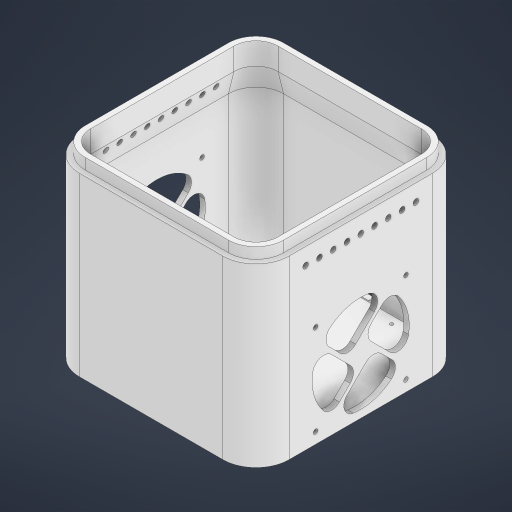
# Autodesk Inventor part: bottom part v2
Saved by Autodesk Inventor 2024.1 (Build 281209000, 209)
## iProperties
Created: 2023-07-11
Part Number: bottom part v2
Material: 일반
Document SubType Name: Modeling
Designer: 6gioc
Density: 1 g/cm^3
Appearance: 기본값
Author: 6gioc
## iProperties of the stored document bottom part v2_3D 인쇄.ipt
Created: 2023-11-02
Part Number: bottom part v2_3D 인쇄
Material: 일반
Document SubType Name: Modeling
Designer: 6gioc
Density: 1 g/cm^3
Appearance: 기본값
Author: 6gioc
Autodesk Inventor part; units mm, degrees
ref_plane "YZ Plane" through (0, 0, 0) normal (1, 0, 0) x (0, 1, 0)
ref_plane "XZ Plane" through (0, 0, 0) normal (0, 1, 0) x (-1, 0, 0)
ref_plane "XY Plane" through (0, 0, 0) normal (0, 0, 1) x (1, 0, 0)
sketch "스케치1" plane through (0, 0, 0) normal (0, 1, 0) x (-1, 0, 0)
  line L0 (-30, 0) -> (-160, 0)
  line L1 (-190, -30) -> (-190, -160)
  line L2 (-160, -190) -> (-30, -190)
  line L3 (0, -160) -> (0, -30)
  arc A0 (-30, -190) -> (0, -160) centre (-30, -160) ccw
  arc A1 (-190, -160) -> (-160, -190) centre (-160, -160) ccw
  arc A2 (-160, 0) -> (-190, -30) centre (-160, -30) ccw
  arc A3 (0, -30) -> (-30, 0) centre (-30, -30) ccw
  line L4 (-30, -185) -> (-160, -185)
  arc A4 (-185, -160) -> (-160, -185) centre (-160, -160) ccw
  line L5 (-185, -160) -> (-185, -30)
  arc A5 (-160, -5) -> (-185, -30) centre (-160, -30) ccw
  line L6 (-160, -5) -> (-30, -5)
  arc A6 (-5, -30) -> (-30, -5) centre (-30, -30) ccw
  line L7 (-5, -30) -> (-5, -160)
  arc A7 (-30, -185) -> (-5, -160) centre (-30, -160) ccw
  point P0 (0, 0)
  point P1 (-190, -190)
  point P2 (-190, 0)
  point P3 (0, -190)
  dimension "d0" = 190
  dimension "d1" = 190
  dimension "d2" = 30
  dimension "d3" = 5
  constraints: 16 end point, 16 point on circle, 8 centre point, 8 point on line, 8 tangent, 4 parallel, 3 equal radius, 2 perpendicular, 1 horizontal, 7 other
  measures "d0" distance of point (0, -190) point (-190, -190)
  measures "d1" distance of point (-190, -190) point (-190, 0)
  measures "d2" radius of A0
  measures "d3" distance between parallel lines of L2 L4
extrude "돌출1" add sketch "스케치1" along normal blind 160
extrude "돌출2" add sketch "스케치1" along normal blind 5 contours L4 A4 L5 A5 L6 A6 L7 A7
sketch "스케치2" plane through (0, 160, 0) normal (0, 1, 0) x (1, 0, 0)
  arc A0 (160, 0) -> (190, 30) centre (160, 30) ccw projected
  line L0 (190, 30) -> (190, 160) projected
  arc A1 (190, 160) -> (160, 190) centre (160, 160) ccw projected
  line L1 (160, 190) -> (30, 190) projected
  arc A2 (30, 190) -> (0, 160) centre (30, 160) ccw projected
  line L2 (0, 160) -> (0, 30) projected
  arc A3 (0, 30) -> (30, 0) centre (30, 30) ccw projected
  line L3 (30, 0) -> (160, 0) projected
  line L4 (5, 30) -> (5, 160) projected
  arc A4 (30, 185) -> (5, 160) centre (30, 160) ccw projected
  line L5 (30, 185) -> (160, 185) projected
  arc A5 (185, 160) -> (160, 185) centre (160, 160) ccw projected
  line L6 (185, 160) -> (185, 30) projected
  arc A6 (160, 5) -> (185, 30) centre (160, 30) ccw projected
  line L7 (160, 5) -> (30, 5) projected
  arc A7 (5, 30) -> (30, 5) centre (30, 30) ccw projected
  line L8 (10, 160) -> (10, 30)
  arc A8 (10, 30) -> (30, 10) centre (30, 30) ccw
  line L9 (30, 10) -> (160, 10)
  arc A9 (160, 10) -> (180, 30) centre (160, 30) ccw
  line L10 (180, 30) -> (180, 160)
  arc A10 (180, 160) -> (160, 180) centre (160, 160) ccw
  line L11 (160, 180) -> (30, 180)
  arc A11 (30, 180) -> (10, 160) centre (30, 160) ccw
  point P0 (0, 0)
  dimension "d8" = 5
  constraints: 8 end point, 8 point on circle, 4 centre point, 7 other
  measures "d8" distance between parallel lines of L4 L8
extrude "돌출3" add sketch "스케치2" along normal blind 10 contours L4 A4 L5 A5 L6 A6 L7 A7
extrude "돌출4" add sketch "스케치2" against normal blind 10 contours L4 A4 L5 A5 L6 A6 L7 A7
chamfer "모따기1" distance 5 distance2 20 8 edges at (95, 150, -5) (177.6777, 150, -12.3223) (185, 150, -95) (177.6777, 150, -177.6777) (95, 150, -185) (12.3223, 150, -177.6777) (5, 150, -95) (12.3223, 150, -12.3223) measured on face at (177.3241, 150, -12.6759) measured on face at (12.6759, 150, -177.3241) measured on face at (12.6759, 150, -12.6759) measured on face at (95, 150, -184.5) measured on face at (184.5, 150, -95) measured on face at (5.5, 150, -95) measured on face at (95, 150, -5.5) measured on face at (177.3241, 150, -177.3241)
sketch "스케치4" plane through (160, 0, -190) normal (0, 0, -1) x (-1, 0, 0)
  line L0 (53, 39.5) -> (77, 39.5)
  line L1 (80, 36.5) -> (80, 9)
  line L2 (77, 6) -> (53, 6)
  line L3 (50, 9) -> (50, 36.5)
  arc A0 (77, 6) -> (80, 9) centre (77, 9) ccw
  arc A1 (50, 9) -> (53, 6) centre (53, 9) ccw
  arc A2 (53, 39.5) -> (50, 36.5) centre (53, 36.5) ccw
  arc A3 (80, 36.5) -> (77, 39.5) centre (77, 36.5) ccw
  line L4 (0, 0) -> (130, 0) projected
  line L5 (130, 0) -> (130, 160) projected
  line L6 (0, 0) -> (0, 160) projected
  circle A4 centre (47.05, 21.1) radius 1.65
  circle A5 centre (82.95, 21.1) radius 1.65
  point P0 (160, 0)
  point P1 (80, 6)
  point P2 (80, 39.5)
  point P3 (50, 6)
  point P4 (50, 22.75)
  dimension "d16" = 30
  dimension "d17" = 33.5
  dimension "d18" = 3
  dimension "d19" = 6
  dimension "d20" = 50
  dimension "d21" = 50
  dimension "d22" = 3.3
  dimension "d23" = 3.3
  dimension "d24" = 15.1
  dimension "d25" = 35.9
  dimension "d26" = 2.95
  constraints: 8 end point, 8 point on circle, 8 tangent, 6 centre point, 6 point on line, 3 equal radius, 2 parallel, 1 horizontal, 1 horizontal alignment, 1 midpoint, 1 perpendicular
  measures "d16" distance of point (80, 6) point (50, 6)
  measures "d17" distance of point (80, 39.5) point (80, 6)
  measures "d18" radius of A0
  measures "d19" distance between parallel lines of L4 L2
  measures "d20" distance between parallel lines of L5 L1
  measures "d21" distance from line of L6 point (50, 22.75)
  measures "d22" diameter of A4
  measures "d23" diameter of A5
  measures "d24" distance from line of L2 A4.centre
  measures "d25" distance of A5.centre A4.centre
  measures "d26" distance from line of L3 A4.centre
extrude "돌출5" cut sketch "스케치4" against normal blind 10
sketch "스케치5" plane through (190, 0, -30) normal (1, 0, 0) x (0, 0, -1)
  circle A0 centre (24, 10) radius 2
  circle A1 centre (106, 10) radius 2
  circle A2 centre (106, 92) radius 2
  circle A3 centre (24, 92) radius 2
  line L0 (19, 97) -> (111, 97)
  line L1 (111, 97) -> (111, 5)
  line L2 (111, 5) -> (19, 5)
  line L3 (19, 5) -> (19, 97)
  line L4 (130, 0) -> (130, 160) projected
  line L5 (0, 0) -> (130, 0) projected
  circle A4 centre (65, 51) radius 44
  circle A5 centre (65, 51) radius 10
  line L6 (24, 92) -> (106, 10)
  line L7 (24, 10) -> (106, 92)
  line L8 (57.9289, 58.0711) -> (88.2274, 88.3696)
  line L9 (72.0711, 58.0711) -> (102.3696, 27.7726)
  line L10 (72.0711, 43.9289) -> (41.7726, 13.6304)
  line L11 (57.9289, 43.9289) -> (27.6304, 74.2274)
  line L12 (60.4038, 46.4038) -> (29.6325, 77.1751)
  line L13 (60.4038, 55.5962) -> (91.1751, 86.3675)
  line L14 (69.5962, 55.5962) -> (100.3675, 24.8249)
  line L15 (69.5962, 46.4038) -> (38.8249, 15.6325)
  circle A6 centre (65, 145) radius 2.5
  line L16 (0, 160) -> (130, 160) projected
  line L17 (130, 130) -> (0, 130) projected
  circle A7 centre (90, 145) radius 2.5
  circle A8 centre (115, 145) radius 2.5
  circle A9 centre (40, 145) radius 2.5
  circle A10 centre (15, 145) radius 2.5
  line L18 (0, 0) -> (0, 160) projected
  circle A11 centre (27.5, 145) radius 2.5
  circle A12 centre (52.5, 145) radius 2.5
  circle A13 centre (77.5, 145) radius 2.5
  circle A14 centre (102.5, 145) radius 2.5
  point P0 (-30, 0)
  point P1 (65.7774, 60.9697)
  point P2 (74.9697, 50.2226)
  point P3 (64.2226, 41.0303)
  point P4 (55.0303, 51.7774)
  point P5 (65, 145)
  dimension "d41" = 88
  dimension "d29" = 4
  dimension "d30" = 4
  dimension "d31" = 4
  dimension "d32" = 4
  dimension "d33" = 82
  dimension "d34" = 82
  dimension "d35" = 92
  dimension "d36" = 92
  dimension "d37" = 5
  dimension "d38" = 5
  dimension "d39" = 19
  dimension "d40" = 5
  dimension "d42" = 20
  dimension "d43" = 3.5
  dimension "d44" = 3.5
  dimension "d45" = 3.5
  dimension "d46" = 3.5
  dimension "d49" = 5
  dimension "d50" = 15
  dimension "d51" = 5
  dimension "d52" = 5
  dimension "d53" = 5
  dimension "d54" = 5
  dimension "d55" = 25
  dimension "d56" = 25
  dimension "d57" = 25
  dimension "d58" = 25
  dimension "d59" = 15
  dimension "d142" = 5
  dimension "d143" = 5
  dimension "d144" = 5
  dimension "d145" = 5
  dimension "d146" = 12.5
  dimension "d147" = 12.5
  dimension "d148" = 12.5
  dimension "d149" = 12.5
  constraints: 28 end point, 14 centre point, 6 horizontal alignment, 6 parallel, 4 perpendicular, 4 point on circle, 4 point on line, 4 tangent, 2 vertical alignment, 1 coincident, 1 horizontal, 21 other
  measures "d29" diameter of A0
  measures "d30" diameter of A1
  measures "d31" diameter of A2
  measures "d32" diameter of A3
  measures "d33" distance of L7.end L6.start
  measures "d34" distance of L7.start L6.start
  measures "d35" distance of L1.end L2.end
  measures "d36" distance of L0.end L1.end
  measures "d37" distance from line of L3 L6.start
  measures "d38" distance from line of L0 L6.start
  measures "d39" distance between parallel lines of L4 L1
  measures "d40" distance between parallel lines of L5 L2
  measures "d42" diameter of A5
  measures "d43" distance between parallel lines of L11 L12
  measures "d44" distance between parallel lines of L8 L13
  measures "d45" distance between parallel lines of L9 L14
  measures "d46" distance between parallel lines of L10 L15
  measures "d49" diameter of A6
  measures "d50" distance from line of L16 A6.centre
  measures "d51" diameter of A7
  measures "d52" diameter of A8
  measures "d53" diameter of A9
  measures "d54" diameter of A10
  measures "d55" distance of A6.centre A9.centre
  measures "d56" distance of A7.centre A6.centre
  measures "d57" distance of A8.centre A7.centre
  measures "d58" distance of A9.centre A10.centre
  measures "d59" distance from line of L18 A10.centre
  measures "d142" diameter of A11
  measures "d143" diameter of A12
  measures "d144" diameter of A13
  measures "d145" diameter of A14
  measures "d146" distance of A9.centre A11.centre
  measures "d147" distance of A12.centre A9.centre
  measures "d148" distance of A13.centre A6.centre
  measures "d149" distance of A8.centre A14.centre
extrude "돌출6" cut sketch "스케치5" against normal blind 5 contours A0 | A1 | A2 | A3 | A4 L7 A5 L13 | L8 L6 A4 | A4 L9 L7 | L6 A5 L12 A4 | L11 L7 A4 | A5 L15 A4 L7 | A4 L6 A5 L14 | A4 L10 L6
extrude "돌출7" cut sketch "스케치5" against normal blind 241.25 contours A6 | A7 | A8 | A9 | A10 | A11 | A12 | A13 | A14
sketch "스케치6" plane through (0, 0, -160) normal (-1, 0, 0) x (0, 0, 1)
  circle A0 centre (24, 10) radius 2
  circle A1 centre (106, 10) radius 2
  circle A2 centre (106, 92) radius 2
  circle A3 centre (24, 92) radius 2
  line L0 (19, 97) -> (111, 97)
  line L1 (111, 97) -> (111, 5)
  line L2 (111, 5) -> (19, 5)
  line L3 (19, 5) -> (19, 97)
  circle A4 centre (65, 51) radius 44
  circle A5 centre (65, 51) radius 10
  line L4 (24, 92) -> (106, 10)
  line L5 (24, 10) -> (106, 92)
  line L6 (57.9289, 58.0711) -> (88.2274, 88.3696)
  line L7 (72.0711, 58.0711) -> (102.3696, 27.7726)
  line L8 (72.0711, 43.9289) -> (41.7726, 13.6304)
  line L9 (57.9289, 43.9289) -> (27.6304, 74.2274)
  line L10 (65.7774, 60.9697) -> (91.1751, 86.3675)
  line L11 (87.4105, 64.2181) -> (38.8249, 15.6325)
  line L12 (55.0303, 51.7774) -> (29.6325, 77.1751)
  line L13 (130, 0) -> (130, 160) projected
  line L14 (0, 0) -> (130, 0) projected
  line L15 (69.5962, 55.5962) -> (100.3675, 24.8249)
  point P0 (160, 0)
  point P1 (80.7926, 9.9318)
  point P2 (64.2226, 41.0303)
  point P3 (74.9697, 50.2226)
  dimension "d72" = 88
  dimension "d62" = 4
  dimension "d63" = 4
  dimension "d64" = 4
  dimension "d65" = 4
  dimension "d66" = 82
  dimension "d67" = 82
  dimension "d68" = 92
  dimension "d69" = 92
  dimension "d70" = 5
  dimension "d71" = 5
  dimension "d73" = 20
  dimension "d75" = 3.5
  dimension "d77" = 3.5
  dimension "d78" = 3.5
  dimension "d79" = 19
  dimension "d80" = 5
  dimension "d81" = 3.5
  constraints: 28 end point, 6 parallel, 6 point on circle, 5 centre point, 4 perpendicular, 4 point on line, 4 tangent, 2 horizontal alignment, 2 vertical alignment, 1 coincident, 1 horizontal, 11 other
  measures "d62" diameter of A0
  measures "d63" diameter of A1
  measures "d64" diameter of A2
  measures "d65" diameter of A3
  measures "d66" distance of L5.end L4.start
  measures "d67" distance of L5.start L4.start
  measures "d68" distance of L1.end L3.start
  measures "d69" distance of L0.end L1.end
  measures "d70" distance from line of L3 L4.start
  measures "d71" distance from line of L0 L4.start
  measures "d73" diameter of A5
  measures "d75" distance between parallel lines of L6 L10
  measures "d77" distance between parallel lines of L8 L11
  measures "d78" distance between parallel lines of L9 L12
  measures "d79" distance between parallel lines of L13 L1
  measures "d80" distance between parallel lines of L14 L2
  measures "d81" distance between parallel lines of L7 L15
extrude "돌출8" cut sketch "스케치6" against normal blind 5 contours A0 | A1 | A2 | A3 | A4 L5 A5 L10 | L6 L4 A4 | A4 L7 L5 | L4 A5 L12 A4 | L9 L5 A4 | A5 L11 A4 L5 | A4 L4 A5 L15 | L4 A4 L8
sketch "스케치7" plane through (0, 0, 0) normal (0, -1, 0) x (1, 0, 0)
  circle A0 centre (135, -178) radius 1.5
  line L0 (160, -190) -> (30, -190) projected
  circle A1 centre (135, -104.3) radius 1.5
  circle A2 centre (147, -92.3) radius 1.5
  line L1 (190, -30) -> (190, -160) projected
  circle A3 centre (53, -178) radius 1.5
  circle A4 centre (53, -104.3) radius 1.5
  circle A5 centre (65, -92.3) radius 1.5
  line L2 (0, -160) -> (0, -30) projected
  point P0 (0, 0)
  dimension "d84" = 3
  dimension "d85" = 12
  dimension "d86" = 3
  dimension "d87" = 73.7
  dimension "d88" = 3
  dimension "d89" = 12
  dimension "d90" = 12
  dimension "d91" = 55
  dimension "d94" = 3
  dimension "d95" = 3
  dimension "d96" = 3
  dimension "d97" = 12
  dimension "d98" = 12
  dimension "d99" = 73.7
  dimension "d100" = 65
  constraints: 6 centre point, 2 vertical alignment, 1 horizontal alignment
  measures "d84" diameter of A0
  measures "d85" distance from line of L0 A0.centre
  measures "d86" diameter of A1
  measures "d87" distance of A1.centre A0.centre
  measures "d88" diameter of A2
  measures "d89" horizontal distance of A2.centre A1.centre
  measures "d90" horizontal distance of A2.centre A1.centre
  measures "d91" distance from line of L1 A0.centre
  measures "d94" diameter of A3
  measures "d95" diameter of A4
  measures "d96" diameter of A5
  measures "d97" horizontal distance of A4.centre A5.centre
  measures "d98" horizontal distance of A5.centre A4.centre
  measures "d99" distance of A4.centre A3.centre
  measures "d100" distance from line of L2 A5.centre
extrude "돌출9" cut sketch "스케치7" against normal blind 5
sketch "스케치9" plane through (0, 5, 0) normal (0, 1, 0) x (1, 0, 0)
  line L0 (185, 160) -> (185, 30) projected
  line L1 (185, 45) -> (5, 45)
  line L2 (5, 30) -> (5, 160) projected
  line L3 (185, 45) -> (365, 45) construction
  circle A0 centre (65, 92.3) radius 1.5 projected
  circle A1 centre (147, 92.3) radius 1.5 projected
  circle A2 centre (53, 104.3) radius 1.5 projected
  circle A3 centre (135, 178) radius 1.5 projected
  circle A4 centre (135, 104.3) radius 1.5 projected
  circle A5 centre (53, 178) radius 1.5 projected
  line L4 (160, 5) -> (30, 5) projected
  arc A6 (160, 5) -> (185, 30) centre (160, 30) ccw projected
  line L5 (185, 160) -> (185, 30) projected
  arc A7 (185, 160) -> (160, 185) centre (160, 160) ccw projected
  line L6 (30, 185) -> (160, 185) projected
  arc A8 (30, 185) -> (5, 160) centre (30, 160) ccw projected
  line L7 (5, 30) -> (5, 160) projected
  arc A9 (5, 30) -> (30, 5) centre (30, 30) ccw projected
  circle A10 centre (180, 40) radius 1.5
  circle A11 centre (180, 40) radius 2.5
  circle A12 centre (180, 27) radius 2.5
  circle A13 centre (163, 10) radius 1.5
  circle A14 centre (163, 10) radius 2.5
  line L8 (95, 45) -> (95, 5)
  circle A15 centre (95, 10) radius 2.5
  circle A16 centre (95, 40) radius 2.5
  circle A17 centre (137.5, 40) radius 2.5
  circle A18 centre (10, 40) radius 1.5
  circle A19 centre (10, 40) radius 2.5
  circle A20 centre (10, 27) radius 2.5
  circle A21 centre (27, 10) radius 1.5
  circle A22 centre (27, 10) radius 2.5
  circle A23 centre (52.5, 40) radius 2.5
  point P0 (0, 0)
  dimension "d108" = 180
  dimension "d109" = 40
  dimension "d110" = 3
  dimension "d111" = 5
  dimension "d112" = 5
  dimension "d113" = 3
  dimension "d114" = 5
  dimension "d115" = 5
  dimension "d116" = 5
  dimension "d117" = 5
  dimension "d118" = 5
  dimension "d119" = 5
  dimension "d121" = 5
  dimension "d122" = 3
  dimension "d123" = 5
  dimension "d124" = 5
  dimension "d125" = 5
  dimension "d126" = 5
  dimension "d127" = 42.5
  dimension "d128" = 85
  dimension "d134" = 3
  constraints: 14 centre point, 6 end point, 6 symmetric about line, 4 coincident, 4 point on line, 2 midpoint, 1 collinear, 1 horizontal, 6 other
  measures "d108" angle of L1 L3
  measures "d109" distance from line of L4 L1.start
  measures "d110" diameter of A10
  measures "d111" diameter of A11
  measures "d112" diameter of A12
  measures "d113" diameter of A13
  measures "d114" diameter of A14
  measures "d115" diameter of A15
  measures "d116" diameter of A16
  measures "d117" distance from line of L4 A15.centre
  measures "d118" distance from line of L1 A16.centre
  measures "d119" distance from line of L4 A14.centre
  measures "d121" distance from line of L0 A12.centre
  measures "d122" vertical distance of L0.end A12.centre
  measures "d123" distance from line of L0 A11.centre
  measures "d124" distance from line of L1 A11.centre
  measures "d125" diameter of A17
  measures "d126" distance from line of L1 A17.centre
  measures "d127" distance of A11.centre A17.centre
  measures "d128" distance from line of L8 A11.centre
  measures "d134" horizontal distance of L4.start A14.centre
extrude "돌출11" add sketch "스케치9" along normal blind 5 contours A16 L8 | L8 A16 | A15 L8 | L8 A15 | A11 | A12 | A14 | A17 | A19 | A20 | A22 | A23
extrude "돌출12" cut sketch "스케치9" against normal blind 5 contours A10 | A13 | A18 | A21
sketch "스케치10" plane through (0, 0, 0) normal (0, -1, 0) x (1, 0, 0)
  circle A0 centre (95, -95) radius 60
  circle A1 centre (95, -95) radius 70
  circle A2 centre (10, -40) radius 1.5 projected
  circle A3 centre (163, -10) radius 1.5 projected
  circle A4 centre (27, -10) radius 1.5 projected
  circle A5 centre (180, -40) radius 1.5 projected
  circle A6 centre (65, -92.3) radius 1.5 projected
  circle A7 centre (147, -92.3) radius 1.5 projected
  circle A8 centre (53, -104.3) radius 1.5 projected
  circle A9 centre (135, -178) radius 1.5 projected
  circle A10 centre (135, -104.3) radius 1.5 projected
  circle A11 centre (53, -178) radius 1.5 projected
  arc A12 (190, -30) -> (160, 0) centre (160, -30) ccw projected
  line L0 (30, 0) -> (160, 0) projected
  arc A13 (30, 0) -> (0, -30) centre (30, -30) ccw projected
  line L1 (0, -160) -> (0, -30) projected
  arc A14 (0, -160) -> (30, -190) centre (30, -160) ccw projected
  line L2 (160, -190) -> (30, -190) projected
  arc A15 (160, -190) -> (190, -160) centre (160, -160) ccw projected
  line L3 (190, -30) -> (190, -160) projected
  point P0 (0, 0)
  point P1 (190, -95)
  point P2 (95, 0)
  dimension "d135" = 120
  dimension "d136" = 140
  constraints: 2 centre point, 2 midpoint, 1 concentric, 1 horizontal alignment, 1 vertical alignment
  measures "d135" diameter of A0
  measures "d136" diameter of A1
extrude "돌출13" add sketch "스케치10" along normal blind 10 contours A1
chamfer "모따기2" distance 10 angle 45 1 edges at (25, 0, -95)
fillet "모깎기1" radius 10 12 edges at (2.5, 86.3675, -68.8249) (2.5, 88.3696, -71.7726) (2.5, 24.8249, -59.6325) (2.5, 15.6325, -121.1751) (2.5, 60.9697, -94.2226) (2.5, 77.1751, -130.3675) (2.5, 74.2274, -132.3696) (2.5, 41.0303, -95.7774) (2.5, 51.7774, -104.9697) (2.5, 50.2226, -85.0303) (2.5, 13.6304, -118.2274) (2.5, 27.7726, -57.6304)
fillet "모깎기2" radius 10 12 edges at (187.5, 15.6325, -68.8249) (187.5, 51.7774, -85.0303) (187.5, 60.9697, -95.7774) (187.5, 41.0303, -94.2226) (187.5, 50.2226, -104.9697) (187.5, 13.6304, -71.7726) (187.5, 74.2274, -57.6304) (187.5, 77.1751, -59.6325) (187.5, 88.3696, -118.2274) (187.5, 86.3675, -121.1751) (187.5, 27.7726, -132.3696) (187.5, 24.8249, -130.3675)
chamfer "모따기3" distance 5 angle 45 10 edges at (92.5, 5, -10) (24.5, 5, -10) (92.5, 5, -40) (50, 5, -40) (7.5, 5, -27) (7.5, 5, -40) (177.5, 5, -40) (177.5, 5, -27) (160.5, 5, -10) (135, 5, -40)
chamfer "모따기4" distance 5 distance2 10 1 edges at (35, 0, -95) measured on face at (35.5, 0, -95)
sketch "스케치11" plane through (95, -10, -95) normal (0, -1, 0) x (1, 0, 0)
  circle A0 centre (0, 0) radius 70 projected
  circle A1 centre (0, 0) radius 60 projected
  circle A2 centre (0, 0) radius 67.5
  circle A3 centre (0, 0) radius 62.5
  point P0 (-95, 95)
  dimension "d158" = 2.5
  dimension "d159" = 2.5
  constraints: 2 centre point
  measures "d158" radial gap between concentric circles of A0 A2
  measures "d159" radial gap between concentric circles of A1 A3
extrude "돌출14" cut sketch "스케치11" against normal blind 5 contours A2
fillet "모깎기3" radius 2.5 2 edges at (27.5, -5, -95) (32.5, -5, -95)
